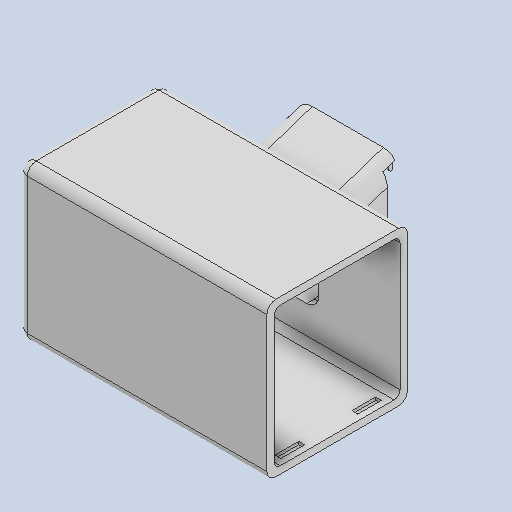
# Autodesk Inventor part: Baterie
Saved by Autodesk Inventor 2025.2 (Build 292293000, 293)
## iProperties
Created: 2024-04-23
Part Number: Baterie
Material: Generic
Document SubType Name: Modeling
Designer: mirun
Density: 1 g/cm^3
Appearance: Default
Author: mirun
Autodesk Inventor part; units mm, degrees
sketch "Sketch1" plane through (0, 0, 0) normal (0, 1, 0) x (-1, 0, 0)
  line L0 (-40.75, 21.25) -> (40.75, 21.25)
  line L1 (40.75, 21.25) -> (40.75, -21.25)
  line L2 (40.75, -21.25) -> (-40.75, -21.25)
  line L3 (-40.75, -21.25) -> (-40.75, 21.25)
  line L4 (-40.75, 21.25) -> (40.75, -21.25) construction
  line L5 (40.75, 21.25) -> (-40.75, -21.25) construction
  point P0 (0, 0)
  dimension "d0" = 81.5
  dimension "d1" = 42.5
  constraints: 12 end point, 2 midpoint, 2 parallel, 1 horizontal, 1 perpendicular
  measures "d0" distance of L1.end L2.end
  measures "d1" distance of L0.end L1.end
extrude "Extrusion1" add sketch "Sketch1" along normal blind 47
shell "Shell1" thickness 2.5 outward yes removed faces 1 at (40.75, 31.3333, 7.0833)
sketch "Sketch2" plane through (40.75, -2.5, -23.75) normal (0, 0, -1) x (-1, 0, 0)
  line L0 (0, 0) -> (84, 0) construction
  line L1 (84, 0) -> (84, 52) construction
  line L2 (0, 52) -> (84, 52) construction
  line L3 (0, 49.5) -> (0, 2.5) construction
  line L4 (0, 26) -> (84, 26) construction
  line L5 (42, 52) -> (42, 0) construction
  line L6 (54, 41) -> (30, 41)
  line L7 (24.5, 35.5) -> (24.5, 16.5)
  line L8 (30, 11) -> (54, 11)
  line L9 (59.5, 16.5) -> (59.5, 35.5)
  line L10 (59.5, 41) -> (24.5, 11) construction
  line L11 (24.5, 41) -> (59.5, 11) construction
  line L12 (52.5, 38) -> (31.5, 38)
  line L13 (27.5, 34) -> (27.5, 18)
  line L14 (31.5, 14) -> (52.5, 14)
  line L15 (56.5, 18) -> (56.5, 34)
  line L16 (56.5, 38) -> (27.5, 14) construction
  line L17 (27.5, 38) -> (56.5, 14) construction
  arc A0 (52.5, 14) -> (56.5, 18) centre (52.5, 18) ccw
  arc A1 (56.5, 34) -> (52.5, 38) centre (52.5, 34) ccw
  arc A2 (31.5, 38) -> (27.5, 34) centre (31.5, 34) ccw
  arc A3 (27.5, 18) -> (31.5, 14) centre (31.5, 18) ccw
  arc A4 (24.5, 16.5) -> (30, 11) centre (30, 16.5) ccw
  arc A5 (54, 11) -> (59.5, 16.5) centre (54, 16.5) ccw
  arc A6 (59.5, 35.5) -> (54, 41) centre (54, 35.5) ccw
  arc A7 (30, 41) -> (24.5, 35.5) centre (30, 35.5) ccw
  point P0 (40.75, 2.5)
  point P1 (42, 11)
  point P2 (132.8324, 127.2861)
  point P3 (27.5, 26)
  point P4 (42, 14)
  point P5 (42, 26)
  point P6 (42, 26)
  point P7 (42, 26)
  point P8 (42, 26)
  dimension "d5" = 35
  dimension "d6" = 30
  dimension "d7" = 3
  dimension "d8" = 3
  dimension "d9" = 4
  dimension "d10" = 5.5
  constraints: 28 end point, 16 point on circle, 16 point on line, 16 tangent, 13 midpoint, 8 centre point, 6 equal radius, 6 parallel, 2 horizontal, 2 perpendicular
  measures "d5" distance of L11.end L10.end
  measures "d6" distance of L10.end L11.start
  measures "d7" distance of point (42, 11) point (42, 14)
  measures "d8" distance from line of point (27.5, 26) L7
  measures "d9" radius of A0
  measures "d10" radius of A4
sketch "Sketch3" plane through (0, 0, 0) normal (0, 1, 0) x (-1, 0, 0)
  point P0 (0, 0)
ref_plane "Work Plane1" through (40.75, 23.5, -23.75) normal (0, -1, 0) x (-1, 0, 0)
sketch "Sketch4" plane through (40.75, 23.5, -23.75) normal (0, -1, 0) x (-1, 0, 0)
  line L0 (0, 0) -> (84, 0) construction
  line L1 (42, 0) -> (49.278, 29.1038)
  point P0 (40.75, -23.75)
  dimension "d13" = 104.04
  dimension "d14" = 30
  constraints: 2 end point, 1 midpoint
  measures "d13" angle of L0 L1
  measures "d14" distance of L1.start L1.end
sweep "Sweep1" add profiles "Sketch2" path "Sketch4"
extrude "Extrusion2" cut sketch "Sketch2" against normal blind 4 contours A1 L15 A0 L14 A3 L13 A2 L12
ref_plane "Work Plane2" through (-26.028, 14, -52.8538) normal (-1, 0, 0) x (0, 1, 0)
ref_plane "Work Plane3" through (-11.028, 14, -52.8538) normal (-1, 0, 0) x (0, 1, 0)
sketch "Sketch5" plane through (-26.028, 14, -52.8538) normal (-1, 0, 0) x (0, 1, 0)
  line L0 (17.5, 0) -> (1.5, 0) construction
  line L1 (9.5, 0) -> (9.5, -38.1996) construction
  line L2 (22.75, -1) -> (21.75, -1)
  line L3 (22.75, -1) -> (23.75, -1) construction
  line L4 (20.75, -2) -> (20.75, -3) construction
  line L5 (20.75, -3) -> (21.75, -3) construction
  line L6 (22.75, -3) -> (22.75, -1)
  line L7 (17.25, 0) -> (22.75, 0) construction
  line L8 (17.25, 0) -> (1.75, 0) construction
  line L9 (9.5, 0) -> (9.5, -18.1412) construction
  line L10 (-3.75, -1) -> (-2.75, -1)
  line L11 (-3.75, -1) -> (-4.75, -1) construction
  line L12 (-1.75, -2) -> (-1.75, -3) construction
  line L13 (-1.75, -3) -> (-3.75, -3)
  line L14 (-3.75, -3) -> (-3.75, -1)
  line L15 (-3.75, -3) -> (-3.75, -5.5)
  line L16 (-3.75, -5.5) -> (22.75, -5.5)
  line L17 (22.75, -5.5) -> (22.75, -3)
  line L18 (0, 0) -> (19, 0) construction
  line L19 (-3.75, -1) -> (-3.75, 0)
  line L20 (-3.75, 0) -> (22.75, 0)
  line L21 (22.75, -1) -> (22.75, 0)
  line L22 (21.75, -1) -> (20.75, -1)
  line L23 (20.75, -1) -> (20.75, -2)
  line L24 (20.75, -2) -> (21.75, -3)
  line L25 (21.75, -3) -> (22.75, -3)
  line L26 (-2.75, -1) -> (-1.75, -1)
  line L27 (-1.75, -1) -> (-1.75, -2)
  line L28 (-1.75, -2) -> (-2.75, -3)
  point P0 (-14, -52.8538)
  point P1 (44.622, -74.2542)
  point P2 (9.5, 0)
  dimension "d20" = 1
  dimension "d21" = 180
  dimension "d23" = 1
  dimension "d24" = 1
  dimension "d25" = 2
  dimension "d26" = 2.5
  dimension "d27" = 13.25
  dimension "d28" = 13.25
  dimension "d29" = 2
  dimension "d37" = 1
  constraints: 54 end point, 7 symmetric about line, 5 midpoint, 5 perpendicular, 4 vertical, 3 horizontal, 2 collinear, 1 point on line
  measures "d20" distance of L2.start L2.end
  measures "d21" angle of L3 L2
  measures "d23" distance of L4.start L4.end
  measures "d24" distance between parallel lines of L7 L2
  measures "d25" distance between parallel lines of L2 L5
  measures "d26" distance of L13.end L15.end
  measures "d27" distance between parallel lines of L1 L15
  measures "d28" distance between parallel lines of L9 L17
  measures "d29" distance between parallel lines of L6 L4
  measures "d37" distance of L10.end L26.end
extrude "Extrusion3" cut sketch "Sketch5" against normal through all
ref_plane "Work Plane5" through (14.5366, 10.25, -24.6969) normal (-0.9701266, 0, 0.2425992) x (0.2425992, 0, 0.9701266)
extrude "Extrusion5" add sketch "Sketch5" against normal up to surface from surface at -15 contours L6 L25 L24 L23 L22 L2 | L10 L26 L27 L28 L13 L14 surface through (14.5366, 10.25, -24.6969) normal (-0.9701266, 0, 0.2425992)
sketch "Sketch6" plane through (8.8708, 36.75, -47.3538) normal (0, 0, -1) x (-1, 0, 0)
  line L0 (1.6909, -21.25) -> (1.6909, -5.25) construction
  line L1 (-0.1489, -13.25) -> (-0.1489, -5.75)
  arc A0 (5.3511, -0.25) -> (-0.1489, -5.75) centre (5.3511, -5.75) ccw
  line L2 (-0.1489, -26.25) -> (-3.0923, -23.25) construction
  line L3 (18.8717, -8.25) -> (8.9967, -8.25)
  line L4 (15.5234, -23.25) -> (15.5234, -13.25)
  line L5 (18.8717, -6.25) -> (18.8717, -8.25)
  arc A1 (30.5792, -6.8617) -> (25.1909, -0.25) centre (25.1928, -5.75) ccw
  line L6 (30.5792, -6.8617) -> (30.5792, -21.8528)
  line L7 (8.9967, -6.25) -> (8.9967, -8.25)
  line L8 (15.5234, -13.25) -> (-0.1489, -13.25)
  line L9 (18.8717, -6.25) -> (8.9967, -6.25)
  line L10 (16.0234, -26.25) -> (16.0234, -0.25) construction
  line L11 (5.3511, -0.25) -> (25.1909, -0.25)
  line L12 (3.6215, -26.25) -> (-0.1489, -26.25) construction
  line L13 (-3.0923, -23.25) -> (15.5234, -23.25)
  line L14 (31.9663, -13.25) -> (-0.1489, -13.25) construction
  line L15 (25.1909, -26.25) -> (3.6215, -26.25)
  arc A2 (0.1421, -23.0839) -> (3.6215, -26.25) centre (5.2278, -20.9898) ccw
  arc A3 (25.1909, -26.25) -> (30.5792, -21.8528) centre (25.1909, -20.75) ccw
  line L16 (16.0234, -25.25) -> (16.0234, -1.25) construction
  line L17 (1.5234, -13.25) -> (30.5234, -13.25) construction
  line L18 (26.6909, -25.25) -> (5.6909, -25.25) construction
  arc A4 (26.6909, -25.25) -> (30.6909, -21.25) centre (26.6909, -21.25) ccw construction
  line L19 (30.4675, -5.25) -> (30.6909, -21.25) construction
  arc A5 (30.4675, -5.25) -> (26.6909, -1.25) centre (26.4675, -5.2438) ccw construction
  line L20 (5.6909, -1.25) -> (26.6909, -1.25) construction
  arc A6 (5.6909, -1.25) -> (1.6909, -5.25) centre (5.6909, -5.25) ccw construction
  arc A7 (1.6909, -21.25) -> (5.6909, -25.25) centre (5.6909, -21.25) ccw construction
  arc A8 (32.0467, -26.5) -> (33.5234, -22.75) centre (28.0234, -22.75) ccw construction
  line L21 (32.0467, -26.5) -> (0, -26.5) construction
  arc A9 (-1.4766, -22.75) -> (0, -26.5) centre (4.0234, -22.75) ccw construction
  line L22 (-1.4766, -3.75) -> (-1.4766, -22.75) construction
  arc A10 (0, 0) -> (-1.4766, -3.75) centre (4.0234, -3.75) ccw construction
  line L23 (32.0467, 0) -> (0, 0) construction
  arc A11 (33.5234, -3.75) -> (32.0467, 0) centre (28.0234, -3.75) ccw construction
  line L24 (33.5234, -22.75) -> (33.5234, -3.75) construction
  line L25 (26.5234, -5.25) -> (5.5234, -21.25) construction
  line L26 (5.5234, -5.25) -> (26.5234, -21.25) construction
  line L27 (-1.4766, -22.75) -> (-1.4766, -3.75) construction
  point P0 (28.0234, -3.75)
  point P1 (4.0234, -3.75)
  point P2 (4.0234, -22.75)
  point P3 (28.0234, -22.75)
  point P4 (30.5792, -0.25)
  point P5 (30.5792, -26.25)
  point P6 (16.0234, -13.25)
  point P7 (16.0234, -13.25)
  point P8 (19.4967, -7.25)
  point P9 (16.0234, -13.25)
  point P10 (16.0234, -13.25)
  point P11 (30.5792, -13.25)
  point P12 (0.2137, -23.25)
  dimension "d47" = 0.5
  dimension "d48" = 10.4734
  constraints: 52 end point, 24 point on circle, 12 centre point, 7 point on line, 3 midpoint, 1 horizontal, 1 vertical, 6 other
  measures "d47" distance between parallel lines of L4 L16
  measures "d48" distance between parallel lines of L27 L7
extrude "Extrusion6" add sketch "Sketch6" against normal blind 2
fillet "Fillet1" radius 2 8 edges at (0, 0, -21.25) (-40.75, 0, 0) (-40.75, 23.5, -21.25) (0, 47, -21.25) (-40.75, 23.5, 21.25) (-40.75, 47, 0) (0, 47, 21.25) (0, 0, 21.25)
fillet "Fillet2" radius 3 8 edges at (-1.25, -2.5, -23.75) (-1.25, 49.5, -23.75) (-1.25, 49.5, 23.75) (-1.25, -2.5, 23.75) (-43.25, -2.5, 0) (-43.25, 49.5, 0) (-43.25, 23.5, -23.75) (-43.25, 23.5, 23.75)
fillet "Fillet3" radius 3 8 edges at (-17.1391, 36.8891, -23.75) (-18.75, 23.5, -23.75) (-17.1391, 10.1109, -23.75) (-1.25, 8.5, -23.75) (14.6391, 10.1109, -23.75) (16.25, 23.5, -23.75) (14.6391, 36.8891, -23.75) (-1.25, 38.5, -23.75)
sketch "Sketch7" plane through (-38.75, 0, -19.25) normal (0, 1, 0) x (1, 0, 0)
  line L0 (79.5, 0) -> (79.5, -38.5) construction
  line L1 (79.5, -19.25) -> (-11.6091, -19.25) construction
  line L2 (77.5, -2.25) -> (75.5, -2.25)
  line L3 (75.5, -2.25) -> (75.5, -10.25)
  line L4 (75.5, -10.25) -> (77.5, -10.25)
  line L5 (77.5, -10.25) -> (77.5, -2.25)
  line L6 (77.5, -36.25) -> (75.5, -36.25)
  line L7 (75.5, -36.25) -> (75.5, -28.25)
  line L8 (75.5, -28.25) -> (77.5, -28.25)
  line L9 (77.5, -28.25) -> (77.5, -36.25)
  point P0 (38.75, -19.25)
  dimension "d49" = 2
  dimension "d50" = 8
  dimension "d51" = 2
  dimension "d52" = 9
  constraints: 18 end point, 4 symmetric about line, 2 horizontal, 2 parallel, 1 midpoint, 1 perpendicular
  measures "d49" distance of L4.end L3.end
  measures "d50" distance of L3.end L2.end
  measures "d51" distance between parallel lines of L0 L5
  measures "d52" distance between parallel lines of L1 L4
extrude "Extrusion7" cut sketch "Sketch7" against normal blind 1
mirror "Mirror1" about plane through (40.75, 23.5, -23.75) normal (0, -1, 0) of "Extrusion7"
body "Solid1"
